Autodesk Fusion 360 part; units mm, degrees
(part 2 of 2)
sketch "Sketch7" plane through (0, 0, -11) normal (0, 0, -1) x (1, 0, 0)
  line L0 (273.1775, 60.5305) -> (273.1775, 7.8909)
  arc A0 (259.7, 5.47) -> (273.1775, 7.8909) centre (226.8375, 227.1492) ccw
  line L1 (259.7, 5.47) -> (259.7, 9.189)
  line L2 (259.7, 9.189) -> (254.65, 9.189)
  line L3 (254.65, 9.189) -> (254.65, 4.78)
  arc A1 (226.8375, 3.0475) -> (254.65, 4.78) centre (226.8375, 227.1492) ccw
  line L4 (226.8375, 3.0475) -> (183.5, 3.0475)
  line L5 (183.5, 3.0475) -> (183.5, 7.2444)
  line L6 (183.5, 7.2444) -> (178.45, 7.2444)
  line L7 (178.45, 7.2444) -> (178.45, 3.0475)
  line L8 (178.45, 3.0475) -> (142.2166, 3.0475)
  line L9 (142.2166, 3.0475) -> (142.2166, 64.9159)
  arc A2 (143.1253, 74.8239) -> (142.2166, 64.9159) centre (196.6857, 64.9159) ccw
  line L10 (143.1253, 74.8239) -> (145.8174, 74.0025)
  line L11 (145.8174, 74.0025) -> (147.0597, 78.0742)
  line L12 (147.0597, 78.0742) -> (144.0657, 78.9877)
  arc A3 (146.683, 86.517) -> (144.0657, 78.9877) centre (196.6857, 64.9159) ccw
  line L13 (146.683, 86.517) -> (153.0767, 101.3175)
  line L14 (153.0767, 101.3175) -> (165.3568, 96.0125)
  line L15 (165.3568, 96.0125) -> (207.025, 96.0125)
  line L16 (207.025, 96.0125) -> (207.025, 92.3887)
  line L17 (207.025, 92.3887) -> (212.075, 92.3887)
  line L18 (212.075, 92.3887) -> (212.075, 96.0125)
  line L19 (212.075, 96.0125) -> (225.5525, 96.0125)
  line L20 (225.5525, 96.0125) -> (225.5525, 79.058)
  line L21 (225.5525, 79.058) -> (273.1775, 79.058)
  line L22 (273.1775, 79.058) -> (273.1775, 65.5805)
  line L23 (273.1775, 65.5805) -> (269.2916, 65.5805)
  line L24 (269.2916, 65.5805) -> (269.2916, 60.5305)
  line L25 (269.2916, 60.5305) -> (273.1775, 60.5305)
  line L26 (228.575, 82.0805) -> (228.575, 99.035)
  line L27 (228.575, 99.035) -> (165.9817, 99.035)
  line L28 (165.9817, 99.035) -> (151.5008, 105.2907)
  line L29 (151.5008, 105.2907) -> (143.9083, 87.7156)
  arc A4 (143.9083, 87.7156) -> (139.1942, 64.9159) centre (196.6857, 64.9159) ccw
  line L30 (139.1942, 64.9159) -> (139.1942, 0.025)
  line L31 (139.1942, 0.025) -> (226.8375, 0.025)
  arc A5 (226.8375, 0.025) -> (276.2, 5.454) centre (226.8375, 227.1492) ccw
  line L32 (276.2, 5.454) -> (276.2, 82.0805)
  line L33 (276.2, 82.0805) -> (228.575, 82.0805)
  line L34 (152.2829, 103.3189) -> (145.2853, 87.1207)
  arc A6 (145.2853, 87.1207) -> (140.6942, 64.9159) centre (196.6857, 64.9159) ccw
  line L35 (140.6942, 64.9159) -> (140.6942, 1.525)
  line L36 (140.6942, 1.525) -> (226.8375, 1.525)
  arc A7 (226.8375, 1.525) -> (274.7, 6.6601) centre (226.8375, 227.1492) ccw
  line L37 (274.7, 6.6601) -> (274.7, 80.5805)
  line L38 (274.7, 80.5805) -> (227.075, 80.5805)
  line L39 (227.075, 80.5805) -> (227.075, 97.535)
  line L40 (227.075, 97.535) -> (165.6716, 97.535)
  line L41 (165.6716, 97.535) -> (152.2829, 103.3189)
  dimension "d42" = -1.5
extrude "Extrude6" add sketch "Sketch7" along normal blind 1.5 contours L26 L27 L28 L29 A4 L30 L31 A5 L32 L33 bodies 1
sketch "Sketch8" plane through (0, -1.725, 0) normal (0, -1, 0) x (1, 0, 0)
  line L0 (178.45, -3.5) -> (178.45, 0)
  line L1 (178.45, 0) -> (140.8942, 0)
  line L2 (140.8942, 0) -> (140.8942, -3.5)
  line L3 (140.8942, -3.5) -> (178.45, -3.5)
  line L4 (155.8942, -2) -> (146.8942, -2)
  line L5 (146.8942, -2) -> (146.8942, -5.5)
  line L6 (146.8942, -5.5) -> (155.8942, -5.5)
  line L7 (155.8942, -5.5) -> (155.8942, -2)
  line L8 (151.3942, -2) -> (151.3942, -17.7481) construction
  circle A0 centre (151.3942, -8.3441) radius 1.35
  dimension "d45" = 9
  dimension "d46" = 3.5
  dimension "d47" = 2
  dimension "d48" = 6
  dimension "d49" = 2.7
  constraint horizontal L4
  constraint vertical L5
  constraint horizontal L6
  constraint vertical L7
  constraint midpoint L4 L8.start
  constraint perpendicular L4 L8
  constraint coincident L8 A0.centre
  measures "d45" distance of L4.start L4.end
  measures "d46" distance of L4.start L6.end
  measures "d47" distance of L1 L4
  measures "d48" distance of L2 L5
  measures "d49" diameter of A0
extrude "Extrude7" cut sketch "Sketch8" along normal blind 8 and the other way blind 12 contours L3 L5 L6 L7 | L3 L4 L5 L7 | A0 bodies 1
fillet "Fillet4" radius 1.75 4 edges at (146.8942, -0.875, -2) (155.8942, -0.875, -2) (155.8942, -1.0513, -5.5) (146.8942, -1.0513, -5.5) on bodies 1
sketch "Sketch9" plane through (0, 0, 0) normal (0, 0, -1) x (1, 0, 0)
  line L0 (269.2916, 60.5305) -> (269.2916, 65.5805)
  line L1 (269.2916, 65.5805) -> (260.2, 65.5805)
  arc A0 (259.7, 66.0805) -> (260.2, 65.5805) centre (260.2, 66.0805) ccw
  line L2 (259.7, 66.0805) -> (259.7, 79.0805)
  arc A1 (260.2, 79.5805) -> (259.7, 79.0805) centre (260.2, 79.0805) ccw
  line L3 (260.2, 79.5805) -> (273.2, 79.5805)
  arc A2 (273.7, 79.0805) -> (273.2, 79.5805) centre (273.2, 79.0805) ccw
  line L4 (273.7, 79.0805) -> (273.7, 66.0805)
  arc A3 (273.2, 65.5805) -> (273.7, 66.0805) centre (273.2, 66.0805) ccw
  line L5 (273.2, 65.5805) -> (274.5, 65.5805)
  line L6 (274.5, 65.5805) -> (274.5, 80.3805)
  line L7 (274.5, 80.3805) -> (226.875, 80.3805)
  line L8 (226.875, 80.3805) -> (226.875, 97.335)
  line L9 (226.875, 97.335) -> (212.075, 97.335)
  line L10 (212.075, 97.335) -> (212.075, 94.7015)
  arc A4 (212.575, 95.2015) -> (212.075, 94.7015) centre (212.575, 94.7015) ccw
  line L11 (212.575, 95.2015) -> (225.575, 95.2015)
  arc A5 (226.075, 94.7015) -> (225.575, 95.2015) centre (225.575, 94.7015) ccw
  line L12 (226.075, 94.7015) -> (226.075, 81.7015)
  arc A6 (225.575, 81.2015) -> (226.075, 81.7015) centre (225.575, 81.7015) ccw
  line L13 (225.575, 81.2015) -> (212.575, 81.2015)
  arc A7 (212.075, 81.7015) -> (212.575, 81.2015) centre (212.575, 81.7015) ccw
  line L14 (212.075, 81.7015) -> (212.075, 92.3887)
  line L15 (212.075, 92.3887) -> (207.025, 92.3887)
  line L16 (207.025, 92.3887) -> (207.025, 81.7015)
  arc A8 (206.525, 81.2015) -> (207.025, 81.7015) centre (206.525, 81.7015) ccw
  line L17 (206.525, 81.2015) -> (193.525, 81.2015)
  arc A9 (193.025, 81.7015) -> (193.525, 81.2015) centre (193.525, 81.7015) ccw
  line L18 (193.025, 81.7015) -> (193.025, 94.7015)
  arc A10 (193.525, 95.2015) -> (193.025, 94.7015) centre (193.525, 94.7015) ccw
  line L19 (193.525, 95.2015) -> (206.525, 95.2015)
  arc A11 (207.025, 94.7015) -> (206.525, 95.2015) centre (206.525, 94.7015) ccw
  line L20 (207.025, 94.7015) -> (207.025, 97.335)
  line L21 (207.025, 97.335) -> (165.6302, 97.335)
  line L22 (165.6302, 97.335) -> (152.3872, 103.056)
  line L23 (152.3872, 103.056) -> (145.4689, 87.0414)
  arc A12 (145.4689, 87.0414) -> (142.8001, 79.3739) centre (196.6857, 64.9159) ccw
  line L24 (142.8001, 79.3739) -> (147.0597, 78.0742)
  line L25 (147.0597, 78.0742) -> (145.8174, 74.0025)
  line L26 (145.8174, 74.0025) -> (141.8525, 75.2122)
  arc A13 (141.8525, 75.2122) -> (140.8942, 64.9159) centre (196.6857, 64.9159) ccw
  line L27 (140.8942, 64.9159) -> (140.8942, 1.725)
  line L28 (140.8942, 1.725) -> (178.45, 1.725)
  line L29 (178.45, 1.725) -> (178.45, 6.835)
  arc A14 (177.95, 6.335) -> (178.45, 6.835) centre (177.95, 6.835) ccw
  line L30 (177.95, 6.335) -> (164.95, 6.335)
  arc A15 (164.45, 6.835) -> (164.95, 6.335) centre (164.95, 6.835) ccw
  line L31 (164.45, 6.835) -> (164.45, 19.835)
  arc A16 (164.95, 20.335) -> (164.45, 19.835) centre (164.95, 19.835) ccw
  line L32 (164.95, 20.335) -> (177.95, 20.335)
  arc A17 (178.45, 19.835) -> (177.95, 20.335) centre (177.95, 19.835) ccw
  line L33 (178.45, 19.835) -> (178.45, 7.2444)
  line L34 (178.45, 7.2444) -> (183.5, 7.2444)
  line L35 (183.5, 7.2444) -> (183.5, 17.168)
  arc A18 (184, 17.668) -> (183.5, 17.168) centre (184, 17.168) ccw
  line L36 (184, 17.668) -> (197, 17.668)
  arc A19 (197.5, 17.168) -> (197, 17.668) centre (197, 17.168) ccw
  line L37 (197.5, 17.168) -> (197.5, 4.168)
  arc A20 (197, 3.668) -> (197.5, 4.168) centre (197, 4.168) ccw
  line L38 (197, 3.668) -> (184, 3.668)
  arc A21 (183.5, 4.168) -> (184, 3.668) centre (184, 4.168) ccw
  line L39 (183.5, 4.168) -> (183.5, 1.725)
  line L40 (183.5, 1.725) -> (226.8375, 1.725)
  arc A22 (226.8375, 1.725) -> (254.65, 3.4473) centre (226.8375, 227.1492) ccw
  line L41 (254.65, 3.4473) -> (254.65, 7.7875)
  arc A23 (254.15, 7.2875) -> (254.65, 7.7875) centre (254.15, 7.7875) ccw
  line L42 (254.15, 7.2875) -> (241.15, 7.2875)
  arc A24 (240.65, 7.7875) -> (241.15, 7.2875) centre (241.15, 7.7875) ccw
  line L43 (240.65, 7.7875) -> (240.65, 20.7875)
  arc A25 (241.15, 21.2875) -> (240.65, 20.7875) centre (241.15, 20.7875) ccw
  line L44 (241.15, 21.2875) -> (254.15, 21.2875)
  arc A26 (254.65, 20.7875) -> (254.15, 21.2875) centre (254.15, 20.7875) ccw
  line L45 (254.65, 20.7875) -> (254.65, 9.189)
  line L46 (254.65, 9.189) -> (259.7, 9.189)
  line L47 (259.7, 9.189) -> (259.7, 21.9305)
  arc A27 (260.2, 22.4305) -> (259.7, 21.9305) centre (260.2, 21.9305) ccw
  line L48 (260.2, 22.4305) -> (273.2, 22.4305)
  arc A28 (273.7, 21.9305) -> (273.2, 22.4305) centre (273.2, 21.9305) ccw
  line L49 (273.7, 21.9305) -> (273.7, 8.9305)
  arc A29 (273.2, 8.4305) -> (273.7, 8.9305) centre (273.2, 8.9305) ccw
  line L50 (273.2, 8.4305) -> (260.2, 8.4305)
  arc A30 (259.7, 8.9305) -> (260.2, 8.4305) centre (260.2, 8.9305) ccw
  line L51 (259.7, 8.9305) -> (259.7, 4.1332)
  arc A31 (259.7, 4.1332) -> (274.5, 6.8214) centre (226.8375, 227.1492) ccw
  line L52 (274.5, 6.8214) -> (274.5, 60.5305)
  line L53 (274.5, 60.5305) -> (273.2, 60.5305)
  arc A32 (273.7, 60.0305) -> (273.2, 60.5305) centre (273.2, 60.0305) ccw
  line L54 (273.7, 60.0305) -> (273.7, 47.0305)
  arc A33 (273.2, 46.5305) -> (273.7, 47.0305) centre (273.2, 47.0305) ccw
  line L55 (273.2, 46.5305) -> (260.2, 46.5305)
  arc A34 (259.7, 47.0305) -> (260.2, 46.5305) centre (260.2, 47.0305) ccw
  line L56 (259.7, 47.0305) -> (259.7, 60.0305)
  arc A35 (260.2, 60.5305) -> (259.7, 60.0305) centre (260.2, 60.0305) ccw
  line L57 (260.2, 60.5305) -> (269.2916, 60.5305)
  line L58 (151.218, 98.3323) -> (164.0701, 92.7802)
  line L59 (164.0701, 92.7802) -> (158.518, 79.9282)
  line L60 (158.518, 79.9282) -> (145.666, 85.4803)
  line L61 (145.666, 85.4803) -> (151.218, 98.3323)
  arc A36 (173.975, 83.035) -> (174.475, 82.535) centre (174.475, 83.035) ccw
  line L62 (173.975, 83.035) -> (173.975, 96.035)
  arc A37 (174.475, 96.535) -> (173.975, 96.035) centre (174.475, 96.035) ccw
  line L63 (174.475, 96.535) -> (187.475, 96.535)
  arc A38 (187.975, 96.035) -> (187.475, 96.535) centre (187.475, 96.035) ccw
  line L64 (187.975, 96.035) -> (187.975, 83.035)
  arc A39 (187.475, 82.535) -> (187.975, 83.035) centre (187.475, 83.035) ccw
  line L65 (187.475, 82.535) -> (174.475, 82.535)
  arc A40 (202.55, 60.175) -> (203.05, 59.675) centre (203.05, 60.175) ccw
  line L66 (202.55, 60.175) -> (202.55, 73.175)
  arc A41 (203.05, 73.675) -> (202.55, 73.175) centre (203.05, 73.175) ccw
  line L67 (203.05, 73.675) -> (216.05, 73.675)
  arc A42 (216.55, 73.175) -> (216.05, 73.675) centre (216.05, 73.175) ccw
  line L68 (216.55, 73.175) -> (216.55, 60.175)
  arc A43 (216.05, 59.675) -> (216.55, 60.175) centre (216.05, 60.175) ccw
  line L69 (216.05, 59.675) -> (203.05, 59.675)
  arc A44 (240.65, 64.9375) -> (241.15, 64.4375) centre (241.15, 64.9375) ccw
  line L70 (240.65, 64.9375) -> (240.65, 77.9375)
  arc A45 (241.15, 78.4375) -> (240.65, 77.9375) centre (241.15, 77.9375) ccw
  line L71 (241.15, 78.4375) -> (254.15, 78.4375)
  arc A46 (254.65, 77.9375) -> (254.15, 78.4375) centre (254.15, 77.9375) ccw
  line L72 (254.65, 77.9375) -> (254.65, 64.9375)
  arc A47 (254.15, 64.4375) -> (254.65, 64.9375) centre (254.15, 64.9375) ccw
  line L73 (254.15, 64.4375) -> (241.15, 64.4375)
  arc A48 (164.45, 63.985) -> (164.95, 63.485) centre (164.95, 63.985) ccw
  line L74 (164.45, 63.985) -> (164.45, 76.985)
  arc A49 (164.95, 77.485) -> (164.45, 76.985) centre (164.95, 76.985) ccw
  line L75 (164.95, 77.485) -> (177.95, 77.485)
  arc A50 (178.45, 76.985) -> (177.95, 77.485) centre (177.95, 76.985) ccw
  line L76 (178.45, 76.985) -> (178.45, 63.985)
  arc A51 (177.95, 63.485) -> (178.45, 63.985) centre (177.95, 63.985) ccw
  line L77 (177.95, 63.485) -> (164.95, 63.485)
  arc A52 (221.6, 61.318) -> (222.1, 60.818) centre (222.1, 61.318) ccw
  line L78 (221.6, 61.318) -> (221.6, 74.318)
  arc A53 (222.1, 74.818) -> (221.6, 74.318) centre (222.1, 74.318) ccw
  line L79 (222.1, 74.818) -> (235.1, 74.818)
  arc A54 (235.6, 74.318) -> (235.1, 74.818) centre (235.1, 74.318) ccw
  line L80 (235.6, 74.318) -> (235.6, 61.318)
  arc A55 (235.1, 60.818) -> (235.6, 61.318) centre (235.1, 61.318) ccw
  line L81 (235.1, 60.818) -> (222.1, 60.818)
  arc A56 (177.95, 44.435) -> (178.45, 44.935) centre (177.95, 44.935) ccw
  line L82 (177.95, 44.435) -> (164.95, 44.435)
  arc A57 (164.45, 44.935) -> (164.95, 44.435) centre (164.95, 44.935) ccw
  line L83 (164.45, 44.935) -> (164.45, 57.935)
  arc A58 (164.95, 58.435) -> (164.45, 57.935) centre (164.95, 57.935) ccw
  line L84 (164.95, 58.435) -> (177.95, 58.435)
  arc A59 (178.45, 57.935) -> (177.95, 58.435) centre (177.95, 57.935) ccw
  line L85 (178.45, 57.935) -> (178.45, 44.935)
  arc A60 (240.65, 45.8875) -> (241.15, 45.3875) centre (241.15, 45.8875) ccw
  line L86 (240.65, 45.8875) -> (240.65, 58.8875)
  arc A61 (241.15, 59.3875) -> (240.65, 58.8875) centre (241.15, 58.8875) ccw
  line L87 (241.15, 59.3875) -> (254.15, 59.3875)
  arc A62 (254.65, 58.8875) -> (254.15, 59.3875) centre (254.15, 58.8875) ccw
  line L88 (254.65, 58.8875) -> (254.65, 45.8875)
  arc A63 (254.15, 45.3875) -> (254.65, 45.8875) centre (254.15, 45.8875) ccw
  line L89 (254.15, 45.3875) -> (241.15, 45.3875)
  arc A64 (183.5, 42.268) -> (184, 41.768) centre (184, 42.268) ccw
  line L90 (183.5, 42.268) -> (183.5, 55.268)
  arc A65 (184, 55.768) -> (183.5, 55.268) centre (184, 55.268) ccw
  line L91 (184, 55.768) -> (197, 55.768)
  arc A66 (197.5, 55.268) -> (197, 55.768) centre (197, 55.268) ccw
  line L92 (197.5, 55.268) -> (197.5, 42.268)
  arc A67 (197, 41.768) -> (197.5, 42.268) centre (197, 42.268) ccw
  line L93 (197, 41.768) -> (184, 41.768)
  line L94 (259.7, 27.9805) -> (259.7, 40.9805)
  arc A68 (260.2, 41.4805) -> (259.7, 40.9805) centre (260.2, 40.9805) ccw
  line L95 (260.2, 41.4805) -> (273.2, 41.4805)
  arc A69 (273.7, 40.9805) -> (273.2, 41.4805) centre (273.2, 40.9805) ccw
  line L96 (273.7, 40.9805) -> (273.7, 27.9805)
  arc A70 (273.2, 27.4805) -> (273.7, 27.9805) centre (273.2, 27.9805) ccw
  line L97 (273.2, 27.4805) -> (260.2, 27.4805)
  arc A71 (259.7, 27.9805) -> (260.2, 27.4805) centre (260.2, 27.9805) ccw
  arc A72 (221.6, 42.268) -> (222.1, 41.768) centre (222.1, 42.268) ccw
  line L98 (221.6, 42.268) -> (221.6, 55.268)
  arc A73 (222.1, 55.768) -> (221.6, 55.268) centre (222.1, 55.268) ccw
  line L99 (222.1, 55.768) -> (235.1, 55.768)
  arc A74 (235.6, 55.268) -> (235.1, 55.768) centre (235.1, 55.268) ccw
  line L100 (235.6, 55.268) -> (235.6, 42.268)
  arc A75 (235.1, 41.768) -> (235.6, 42.268) centre (235.1, 42.268) ccw
  line L101 (235.1, 41.768) -> (222.1, 41.768)
  arc A76 (202.55, 41.125) -> (203.05, 40.625) centre (203.05, 41.125) ccw
  line L102 (202.55, 41.125) -> (202.55, 54.125)
  arc A77 (203.05, 54.625) -> (202.55, 54.125) centre (203.05, 54.125) ccw
  line L103 (203.05, 54.625) -> (216.05, 54.625)
  arc A78 (216.55, 54.125) -> (216.05, 54.625) centre (216.05, 54.125) ccw
  line L104 (216.55, 54.125) -> (216.55, 41.125)
  arc A79 (216.05, 40.625) -> (216.55, 41.125) centre (216.05, 41.125) ccw
  line L105 (216.05, 40.625) -> (203.05, 40.625)
  arc A80 (221.6, 23.218) -> (222.1, 22.718) centre (222.1, 23.218) ccw
  line L106 (221.6, 23.218) -> (221.6, 36.218)
  arc A81 (222.1, 36.718) -> (221.6, 36.218) centre (222.1, 36.218) ccw
  line L107 (222.1, 36.718) -> (235.1, 36.718)
  arc A82 (235.6, 36.218) -> (235.1, 36.718) centre (235.1, 36.218) ccw
  line L108 (235.6, 36.218) -> (235.6, 23.218)
  arc A83 (235.1, 22.718) -> (235.6, 23.218) centre (235.1, 23.218) ccw
  line L109 (235.1, 22.718) -> (222.1, 22.718)
  arc A84 (240.65, 26.8375) -> (241.15, 26.3375) centre (241.15, 26.8375) ccw
  line L110 (240.65, 26.8375) -> (240.65, 39.8375)
  arc A85 (241.15, 40.3375) -> (240.65, 39.8375) centre (241.15, 39.8375) ccw
  line L111 (241.15, 40.3375) -> (254.15, 40.3375)
  arc A86 (254.65, 39.8375) -> (254.15, 40.3375) centre (254.15, 39.8375) ccw
  line L112 (254.65, 39.8375) -> (254.65, 26.8375)
  arc A87 (254.15, 26.3375) -> (254.65, 26.8375) centre (254.15, 26.8375) ccw
  line L113 (254.15, 26.3375) -> (241.15, 26.3375)
  arc A88 (202.55, 22.075) -> (203.05, 21.575) centre (203.05, 22.075) ccw
  line L114 (202.55, 22.075) -> (202.55, 35.075)
  arc A89 (203.05, 35.575) -> (202.55, 35.075) centre (203.05, 35.075) ccw
  line L115 (203.05, 35.575) -> (216.05, 35.575)
  arc A90 (216.55, 35.075) -> (216.05, 35.575) centre (216.05, 35.075) ccw
  line L116 (216.55, 35.075) -> (216.55, 22.075)
  arc A91 (216.05, 21.575) -> (216.55, 22.075) centre (216.05, 22.075) ccw
  line L117 (216.05, 21.575) -> (203.05, 21.575)
  arc A92 (164.45, 25.885) -> (164.95, 25.385) centre (164.95, 25.885) ccw
  line L118 (164.45, 25.885) -> (164.45, 38.885)
  arc A93 (164.95, 39.385) -> (164.45, 38.885) centre (164.95, 38.885) ccw
  line L119 (164.95, 39.385) -> (177.95, 39.385)
  arc A94 (178.45, 38.885) -> (177.95, 39.385) centre (177.95, 38.885) ccw
  line L120 (178.45, 38.885) -> (178.45, 25.885)
  arc A95 (177.95, 25.385) -> (178.45, 25.885) centre (177.95, 25.885) ccw
  line L121 (177.95, 25.385) -> (164.95, 25.385)
  line L122 (183.5, 23.218) -> (183.5, 36.218)
  arc A96 (184, 36.718) -> (183.5, 36.218) centre (184, 36.218) ccw
  line L123 (184, 36.718) -> (197, 36.718)
  arc A97 (197.5, 36.218) -> (197, 36.718) centre (197, 36.218) ccw
  line L124 (197.5, 36.218) -> (197.5, 23.218)
  arc A98 (197, 22.718) -> (197.5, 23.218) centre (197, 23.218) ccw
  line L125 (197, 22.718) -> (184, 22.718)
  arc A99 (183.5, 23.218) -> (184, 22.718) centre (184, 23.218) ccw
  arc A100 (183.5, 61.318) -> (184, 60.818) centre (184, 61.318) ccw
  line L126 (183.5, 61.318) -> (183.5, 74.318)
  arc A101 (184, 74.818) -> (183.5, 74.318) centre (184, 74.318) ccw
  line L127 (184, 74.818) -> (197, 74.818)
  arc A102 (197.5, 74.318) -> (197, 74.818) centre (197, 74.318) ccw
  line L128 (197.5, 74.318) -> (197.5, 61.318)
  arc A103 (197, 60.818) -> (197.5, 61.318) centre (197, 61.318) ccw
  line L129 (197, 60.818) -> (184, 60.818)
  line L130 (145.4, 54.46) -> (145.4, 67.46)
  arc A104 (145.9, 67.96) -> (145.4, 67.46) centre (145.9, 67.46) ccw
  line L131 (145.9, 67.96) -> (158.9, 67.96)
  arc A105 (159.4, 67.46) -> (158.9, 67.96) centre (158.9, 67.46) ccw
  line L132 (159.4, 67.46) -> (159.4, 54.46)
  arc A106 (158.9, 53.96) -> (159.4, 54.46) centre (158.9, 54.46) ccw
  line L133 (158.9, 53.96) -> (145.9, 53.96)
  arc A107 (145.4, 54.46) -> (145.9, 53.96) centre (145.9, 54.46) ccw
  arc A108 (221.6, 4.168) -> (222.1, 3.668) centre (222.1, 4.168) ccw
  line L134 (221.6, 4.168) -> (221.6, 17.168)
  arc A109 (222.1, 17.668) -> (221.6, 17.168) centre (222.1, 17.168) ccw
  line L135 (222.1, 17.668) -> (235.1, 17.668)
  arc A110 (235.6, 17.168) -> (235.1, 17.668) centre (235.1, 17.168) ccw
  line L136 (235.6, 17.168) -> (235.6, 4.168)
  arc A111 (235.1, 3.668) -> (235.6, 4.168) centre (235.1, 4.168) ccw
  line L137 (235.1, 3.668) -> (222.1, 3.668)
  arc A112 (202.55, 3.025) -> (203.05, 2.525) centre (203.05, 3.025) ccw
  line L138 (202.55, 3.025) -> (202.55, 16.025)
  arc A113 (203.05, 16.525) -> (202.55, 16.025) centre (203.05, 16.025) ccw
  line L139 (203.05, 16.525) -> (216.05, 16.525)
  arc A114 (216.55, 16.025) -> (216.05, 16.525) centre (216.05, 16.025) ccw
  line L140 (216.55, 16.025) -> (216.55, 3.025)
  arc A115 (216.05, 2.525) -> (216.55, 3.025) centre (216.05, 3.025) ccw
  line L141 (216.05, 2.525) -> (203.05, 2.525)
  line L142 (157.3942, 37.125) -> (145.3942, 37.125)
  line L143 (145.3942, 37.125) -> (145.3942, 39.125)
  line L144 (145.3942, 39.125) -> (157.3942, 39.125)
  line L145 (157.3942, 39.125) -> (157.3942, 37.125)
  line L146 (151.3942, 37.125) -> (151.3942, 1.725) construction
  line L147 (148.6442, 1.725, 2) -> (154.1442, 1.725, 2) construction
  line L148 (151.3942, 1.725, 2) -> (151.3942, 1.725, 0) construction
  dimension "d56" = 35.4
  constraint horizontal L142
  constraint vertical L143
  constraint horizontal L144
  constraint vertical L145
  constraint midpoint L142 L146.start
  constraint coincident L28 L146.end
  constraint perpendicular L28 L146
  measures "d56" distance of L28 L142
extrude "Extrude8" add sketch "Sketch9" along normal blind 2.5 contours L142 L143 L144 L145 bodies 1
fillet "Fillet5" radius 1 25 edges at (251.6676, -1.3863, 1.5) (183.0158, -0.025, 1.5) (276.2, -43.7673, 1.5) (252.3875, -82.0805, 1.5) (228.575, -90.5577, 1.5) (197.2784, -99.035, 1.5) (158.7412, -102.1629, 1.5) (139.1942, -32.4705, 1.5) (140.385, -76.5569, 1.5) (147.7045, -96.5032, 1.5) (276.2, -5.454, -5.5) (276.2, -82.0805, -5.5) (276.2, -43.7673, -12.5) (183.0158, -0.025, -12.5) (251.6676, -1.3863, -12.5) (139.1942, -0.025, -5.5) (147.7045, -96.5032, -12.5) (140.385, -76.5569, -12.5) (139.1942, -32.4705, -12.5) (151.5008, -105.2907, -5.5) (228.575, -99.035, -5.5) (252.3875, -82.0805, -12.5) (228.575, -90.5577, -12.5) (197.2784, -99.035, -12.5) (158.7412, -102.1629, -12.5) on bodies 1
fillet "Fillet6" radius 1 4 edges at (226.2138, -79.7193, -7.25) (226.875, -80.3805, -1.75) (165.6302, -97.335, -1.75) (165.4935, -96.6738, -7.25) on bodies 1
fillet "Fillet7" radius 0.5 2 edges at (227.075, -80.5805, -11.75) (165.6716, -97.535, -11.75) on bodies 1
fillet "Fillet8" radius 0.75 5 edges at (274.7, -6.6601, -11.75) (140.6942, -1.525, -11.75) (152.2829, -103.3189, -11.75) (227.075, -97.535, -11.75) (274.7, -80.5805, -11.75) on bodies 1
sketch "Sketch10" plane through (0, 0, -11) normal (0, 0, -1) x (1, 0, 0)
  arc A0 (274.7, 79.8305) -> (273.95, 80.5805) centre (273.95, 79.8305) ccw
  line L0 (273.95, 80.5805) -> (227.575, 80.5805)
  arc A1 (227.075, 81.0805) -> (227.575, 80.5805) centre (227.575, 81.0805) ccw
  line L1 (227.075, 81.0805) -> (227.075, 96.785)
  arc A2 (227.075, 96.785) -> (226.325, 97.535) centre (226.325, 96.785) ccw
  line L2 (226.325, 97.535) -> (165.775, 97.535)
  arc A3 (165.5767, 97.576) -> (165.775, 97.535) centre (165.775, 98.035) ccw
  line L3 (165.5767, 97.576) -> (152.9714, 103.0214)
  arc A4 (152.9714, 103.0214) -> (151.9855, 102.6304) centre (152.674, 102.3329) ccw
  line L4 (151.9855, 102.6304) -> (145.2853, 87.1207)
  arc A5 (145.2853, 87.1207) -> (140.6942, 64.9159) centre (196.6857, 64.9159) ccw
  line L5 (140.6942, 64.9159) -> (140.6942, 2.275)
  arc A6 (140.6942, 2.275) -> (141.4442, 1.525) centre (141.4442, 2.275) ccw
  line L6 (141.4442, 1.525) -> (226.8375, 1.525)
  arc A7 (226.8375, 1.525) -> (274.1071, 6.5322) centre (226.8375, 227.1492) ccw
  arc A8 (274.1071, 6.5322) -> (274.7, 7.2655) centre (273.95, 7.2655) ccw
  line L7 (274.7, 7.2655) -> (274.7, 79.8305)
  ellipse E0 centre (165.5668, 97.028) end of major axis (165.361, 96.0329) minor radius 1 (165.1699, 96.0933) -> (165.5604, 96.0125) ccw
  line L8 (165.5604, 96.0125) -> (207.025, 96.0125)
  line L9 (207.025, 96.0125) -> (207.025, 92.3887)
  line L10 (207.025, 92.3887) -> (212.075, 92.3887)
  line L11 (212.075, 92.3887) -> (212.075, 96.0125)
  line L12 (212.075, 96.0125) -> (225.5525, 96.0125)
  line L13 (225.5525, 96.0125) -> (225.5525, 80.0429)
  ellipse E1 centre (226.568, 80.0735) end of major axis (225.8392, 79.3447) minor radius 1 (225.5525, 80.0429) -> (226.5374, 79.058) ccw
  line L14 (226.5374, 79.058) -> (273.1775, 79.058)
  line L15 (273.1775, 79.058) -> (273.1775, 65.5805)
  line L16 (273.1775, 65.5805) -> (269.2916, 65.5805)
  line L17 (269.2916, 65.5805) -> (269.2916, 60.5305)
  line L18 (269.2916, 60.5305) -> (273.1775, 60.5305)
  line L19 (273.1775, 60.5305) -> (273.1775, 7.8909)
  arc A9 (259.7, 5.47) -> (273.1775, 7.8909) centre (226.8375, 227.1492) ccw
  line L20 (259.7, 5.47) -> (259.7, 9.189)
  line L21 (259.7, 9.189) -> (254.65, 9.189)
  line L22 (254.65, 9.189) -> (254.65, 4.78)
  arc A10 (226.8375, 3.0475) -> (254.65, 4.78) centre (226.8375, 227.1492) ccw
  line L23 (226.8375, 3.0475) -> (183.5, 3.0475)
  line L24 (183.5, 3.0475) -> (183.5, 7.2444)
  line L25 (183.5, 7.2444) -> (178.45, 7.2444)
  line L26 (178.45, 7.2444) -> (178.45, 3.0475)
  line L27 (178.45, 3.0475) -> (142.2166, 3.0475)
  line L28 (142.2166, 3.0475) -> (142.2166, 64.9159)
  arc A11 (143.1253, 74.8239) -> (142.2166, 64.9159) centre (196.6857, 64.9159) ccw
  line L29 (143.1253, 74.8239) -> (145.8174, 74.0025)
  line L30 (145.8174, 74.0025) -> (147.0597, 78.0742)
  line L31 (147.0597, 78.0742) -> (144.0657, 78.9877)
  arc A12 (146.683, 86.517) -> (144.0657, 78.9877) centre (196.6857, 64.9159) ccw
  line L32 (146.683, 86.517) -> (153.0767, 101.3175)
  line L33 (153.0767, 101.3175) -> (165.1699, 96.0933)
  arc A13 (165.4974, 97.3924) -> (165.775, 97.335) centre (165.775, 98.035) ccw
  line L34 (226.325, 97.335) -> (165.775, 97.335)
  arc A14 (226.875, 96.785) -> (226.325, 97.335) centre (226.325, 96.785) ccw
  line L35 (226.875, 81.0805) -> (226.875, 96.785)
  arc A15 (226.875, 81.0805) -> (227.575, 80.3805) centre (227.575, 81.0805) ccw
  line L36 (273.95, 80.3805) -> (227.575, 80.3805)
  arc A16 (274.5, 79.8305) -> (273.95, 80.3805) centre (273.95, 79.8305) ccw
  line L37 (274.5, 7.2655) -> (274.5, 79.8305)
  arc A17 (274.0652, 6.7278) -> (274.5, 7.2655) centre (273.95, 7.2655) ccw
  arc A18 (226.8375, 1.725) -> (274.0652, 6.7278) centre (226.8375, 227.1492) ccw
  line L38 (141.4442, 1.725) -> (226.8375, 1.725)
  arc A19 (140.8942, 2.275) -> (141.4442, 1.725) centre (141.4442, 2.275) ccw
  line L39 (140.8942, 64.9159) -> (140.8942, 2.275)
  arc A20 (145.4689, 87.0414) -> (140.8942, 64.9159) centre (196.6857, 64.9159) ccw
  line L40 (152.1691, 102.5511) -> (145.4689, 87.0414)
  arc A21 (152.8921, 102.8378) -> (152.1691, 102.5511) centre (152.674, 102.3329) ccw
  line L41 (165.4974, 97.3924) -> (152.8921, 102.8378)
  circle A22 centre (271.6034, 62.9783) radius 1
  circle A23 centre (209.5928, 94.8476) radius 1
  circle A24 centre (144.4946, 76.6627) radius 1
  circle A25 centre (181, 5) radius 1
  circle A26 centre (257.2701, 6.717) radius 1
  dimension "d67" = -0.2
  dimension "d70" = 2
  dimension "d71" = 2
  dimension "d72" = 2
  dimension "d73" = 2
  dimension "d74" = 2
  measures "d70" diameter of A22
  measures "d71" diameter of A23
  measures "d72" diameter of A24
  measures "d73" diameter of A25
  measures "d74" diameter of A26
extrude "Extrude9" add sketch "Sketch10" along normal blind 1.5 separate body contours E0 L8 L9 L10 L11 L12 L13 E1 L14 L15 L16 L17 L18 L19 A9 L20 L21 L22 A10 L23 L24 L25 L26 L27 L28 A11 L29 L30 L31 A12 L32 L33 | A13 L34 A14 L35 A15 L36 A16 L37 A17 A18 L38 A19 L39 A20 L40 A21 L41 | A22 | A23 | A24 | A25 | A26 makes body 2
extrude "Extrude10" cut sketch "Sketch10" along normal blind -5 and the other way blind -8.5 contours A22 | A23 | A24 | A25 | A26 bodies 1 2
equation "switch_margin = 2.5 mm"
equation "wall_thickness = 1.7 mm"
equation "d8 = switch_margin"
equation "d9 = switch_margin"
equation "d11 = switch_margin"
equation "d12 = switch_margin"
equation "d13 = switch_margin"
equation "d15 = wall_thickness"
equation "d24 = switch_margin"
named bodies: "Shell", "Bottom Plate"
